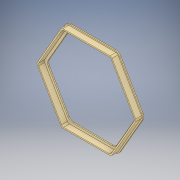
# Autodesk Inventor part: Cover v1
Saved by Autodesk Inventor 2019 (Build 230136000, 136)
## iProperties
Created: 2021-07-14
Part Number: Cover v1
Material: Generic
Document SubType Name: Modeling
Designer: Lix
Density: 1 g/cm^3
Appearance: Beige
Author: Lix
Autodesk Inventor part; units mm, degrees
ref_plane "YZ Plane" through (0, 0, 0) normal (1, 0, 0) x (0, 1, 0)
ref_plane "XZ Plane" through (0, 0, 0) normal (0, 1, 0) x (-1, 0, 0)
ref_plane "XY Plane" through (0, 0, 0) normal (0, 0, 1) x (1, 0, 0)
sketch "Sketch1" plane through (0, 0, 0) normal (0, 0, 1) x (1, 0, 0)
  line L0 (43.3013, -75) -> (-43.3013, -75)
  line L1 (-43.3013, -75) -> (-86.6025, 0)
  line L2 (-86.6025, 0) -> (-43.3013, 75)
  line L3 (-43.3013, 75) -> (43.3013, 75)
  line L4 (43.3013, 75) -> (86.6025, 0)
  line L5 (86.6025, 0) -> (43.3013, -75)
  point P0 (0, 0)
  point P1 (0, 0)
  dimension "d0" = 150
  constraints: 12 end point, 1 coincident, 1 horizontal, 13 other
  measures "d0" distance between parallel lines of L4 L1
extrude "Extrusion1" add sketch "Sketch1" along normal blind 2
sketch "Sketch5" plane through (0, 0, 2) normal (0, 0, 1) x (1, 0, 0)
  line L0 (-43.3013, -75) -> (43.3013, -75) projected
  line L1 (43.3013, -75) -> (86.6025, 0) projected
  line L2 (86.6025, 0) -> (43.3013, 75) projected
  line L3 (43.3013, 75) -> (-43.3013, 75) projected
  line L4 (-43.3013, 75) -> (-86.6025, 0) projected
  line L5 (-86.6025, 0) -> (-43.3013, -75) projected
  line L6 (-84.2931, 0) -> (-42.1466, 73)
  line L7 (-42.1466, 73) -> (42.1466, 73)
  line L8 (42.1466, 73) -> (84.2931, 0)
  line L9 (84.2931, 0) -> (42.1466, -73)
  line L10 (42.1466, -73) -> (-42.1466, -73)
  line L11 (-42.1466, -73) -> (-84.2931, 0)
  line L12 (-81.9837, 0) -> (-40.9919, 71)
  line L13 (-40.9919, 71) -> (40.9919, 71)
  line L14 (40.9919, 71) -> (81.9837, 0)
  line L15 (81.9837, 0) -> (40.9919, -71)
  line L16 (40.9919, -71) -> (-40.9919, -71)
  line L17 (-40.9919, -71) -> (-81.9837, 0)
  point P0 (0, 0)
  dimension "d15" = 2
  dimension "d16" = 2
  constraints: 24 end point, 10 other
  measures "d15" distance between parallel lines of L4 L6
  measures "d16" distance between parallel lines of L11 L17
extrude "Extrusion5" add sketch "Sketch5" along normal blind 10 contours L6 L7 L8 L9 L10 L11
sketch "Sketch7" plane through (0, 0, 2) normal (0, 0, 1) x (1, 0, 0)
  line L0 (40.9919, 71) -> (-40.9919, 71) projected
  line L1 (-40.9919, 71) -> (-81.9837, 0) projected
  line L2 (-81.9837, 0) -> (-40.9919, -71) projected
  line L3 (-40.9919, -71) -> (40.9919, -71) projected
  line L4 (40.9919, -71) -> (81.9837, 0) projected
  line L5 (81.9837, 0) -> (40.9919, 71) projected
  line L6 (-38.6825, -67) -> (-77.3649, 0)
  line L7 (-77.3649, 0) -> (-38.6825, 67)
  line L8 (-38.6825, 67) -> (38.6825, 67)
  line L9 (38.6825, 67) -> (77.3649, 0)
  line L10 (77.3649, 0) -> (38.6825, -67)
  line L11 (38.6825, -67) -> (-38.6825, -67)
  point P0 (0, 0)
  dimension "d19" = 4
  constraints: 12 end point, 5 other
  measures "d19" distance between parallel lines of L2 L6
extrude "Extrusion6" cut sketch "Sketch7" against normal blind 7 contours L6 L7 L8 L9 L10 L11
fillet "Fillet1" radius 10 6 edges at (43.3013, 75, 1) (86.6025, 0, 1) (43.3013, -75, 1) (-43.3013, -75, 1) (-86.6025, 0, 1) (-43.3013, 75, 1)
fillet "Fillet1" radius 4 12 edges at (42.1466, -73, 7) (-40.9919, -71, 7) (-84.2931, 0, 7) (-42.1466, 73, 7) (42.1466, 73, 7) (84.2931, 0, 7) (40.9919, -71, 7) (81.9837, 0, 7) (-40.9919, 71, 7) (40.9919, 71, 7) (-42.1466, -73, 7) (-81.9837, 0, 7)
fillet "Fillet2" radius 10 6 edges at (38.6825, -67, 1) (77.3649, 0, 1) (38.6825, 67, 1) (-38.6825, 67, 1) (-77.3649, 0, 1) (-38.6825, -67, 1)
body "Solid1"
